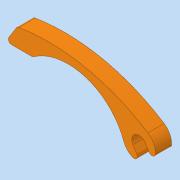
# Autodesk Inventor part: GearMotorMountArm
Saved by Autodesk Inventor 2017.3 (Build 213256000, 256)
## iProperties
Created: 2019-01-08
Part Number: GearMotorMountArm
Material: ABS Plastic
Document SubType Name: Modeling
Designer: Derek Wider
Density: 1.06 g/cm^3
Appearance: Orange
Author: Derek Wider
Autodesk Inventor part; units mm, degrees
ref_plane "YZ Plane" through (0, 0, 0) normal (1, 0, 0) x (0, 1, 0)
ref_plane "XZ Plane" through (0, 0, 0) normal (0, 1, 0) x (-1, 0, 0)
ref_plane "XY Plane" through (0, 0, 0) normal (0, 0, 1) x (1, 0, 0)
sketch "Sketch1" plane through (0, 0, 0) normal (0, 0, 1) x (1, 0, 0)
  circle A0 centre (20.955, -36.2951) radius 47.625 construction
  line L0 (0, 5.1308) -> (17.0942, 5.1308) construction
  arc A1 (43.3585, 0.9173) -> (40.4615, -0.9173) centre (41.91, 0) ccw
  arc A2 (45.1788, -1.9573) -> (42.2818, -3.7918) centre (41.91, 0) ccw
  line L1 (17.0942, 5.1308) -> (10.7442, 5.1308)
  line L2 (10.7442, 5.1308) -> (13.4588, 9.4247)
  arc A3 (43.9676, 3.2066) -> (13.4588, 9.4247) centre (20.6843, -33.0781) ccw
  arc A4 (38.3259, -1.2925) -> (17.0942, 5.1308) centre (25.3195, -5.9828) ccw
  line L3 (43.3585, 0.9173) -> (45.1788, -1.9573)
  line L4 (40.4615, -0.9173) -> (42.2818, -3.7918)
  point P0 (0, 0)
  point P1 (62.865, -36.2951)
  dimension "d0" = 41.91
  dimension "d1" = 95.25
  dimension "d2" = 41.91
  dimension "d3" = 41.91
  dimension "d4" = 5.1308
  dimension "d5" = 17.0942
  dimension "d6" = 3.429
  dimension "d7" = 7.62
  dimension "d8" = 6.35
  dimension "d9" = 5.08
  dimension "d10" = 41.91
  dimension "d11" = 41.91
  constraints: 10 end point, 10 point on circle, 5 centre point, 3 tangent, 2 coincident, 2 parallel, 2 point on line, 1 horizontal, 1 horizontal alignment, 1 vertical alignment
  measures "d0" distance of point (0, 0) point (41.91, 0)
  measures "d1" diameter of A0
  measures "d2" distance of A0.centre point (0, 0)
  measures "d3" distance of A0.centre point (41.91, 0)
  measures "d4" distance from line of L0 point (0, 0)
  measures "d5" distance of L0.start L0.end
  measures "d6" diameter of A1
  measures "d7" diameter of A2
  measures "d8" distance of L0.end L1.end
  measures "d9" distance of L1.end L2.end
  measures "d10" distance of A0.centre point (62.865, -36.295)
  measures "d11" distance of point (62.865, -36.295) A1.centre
extrude "Extrusion1" add sketch "Sketch1" along normal blind 3.81
fillet "Fillet1" radius 0.762 5 edges at (42.2818, -3.7918, 1.905) (45.1788, -1.9573, 1.905) (17.0942, 5.1308, 1.905) (13.4588, 9.4247, 1.905) (10.7442, 5.1308, 1.905)
body "Solid1"
